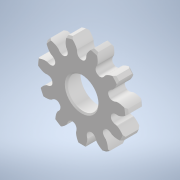
# Autodesk Inventor part: parasit_gear
Saved by Autodesk Inventor 2022 (Build 260153000, 153)
## iProperties
Created: 2024-09-10
Part Number: parasit_gear
Material: Типовые
Document SubType Name: Modeling
Designer: Andrey
Density: 1 g/cm^3
Appearance: По умолчанию
Author: Andrey
Autodesk Inventor part; units mm, degrees
ref_plane "YZ Plane" through (0, 0, 0) normal (1, 0, 0) x (0, 1, 0)
ref_plane "XZ Plane" through (0, 0, 0) normal (0, 1, 0) x (-1, 0, 0)
ref_plane "XY Plane" through (0, 0, 0) normal (0, 0, 1) x (1, 0, 0)
sketch "Эскиз1" plane through (0, 0, 0) normal (0, 0, 1) x (1, 0, 0)
  spline S0 degree 3 poles (-3.0473, 12.5821) (-3.001, 12.5436) (-2.9083, 12.4667) (-2.7729, 12.3469) (-2.6403, 12.2241) (-2.511, 12.0979) (-2.385, 11.9683) (-2.2627, 11.8352) (-2.1444, 11.6986) (-2.0303, 11.5585) (-1.9208, 11.4147) (-1.8163, 11.2672) (-1.7175, 11.1159) (-1.6248, 10.9607) (-1.5393, 10.8014) (-1.462, 10.638) (-1.4063, 10.498) (-1.368, 10.3837) (-1.3532, 10.3253) (-1.3457, 10.2961) knots 0 0 0 0 0.018071 0.036141 0.054212 0.072283 0.090353 0.108424 0.126494 0.144565 0.162635 0.180705 0.198775 0.216845 0.234914 0.252983 0.271051 0.280085 0.289119 0.289119 0.289119 0.289119
  spline S1 degree 3 poles (-1.3457, 10.2961) (-1.3472, 10.2417) (-1.3501, 10.1328) (-1.344, 9.9695) (-1.3289, 9.8068) (-1.3048, 9.6452) (-1.2696, 9.4855) (-1.2292, 9.3555) (-1.1924, 9.2529) (-1.1592, 9.1783) (-1.1249, 9.1042) (-1.0848, 9.033) (-1.042, 8.9634) (-0.9953, 8.8964) (-0.9441, 8.8326) (-0.8892, 8.7721) (-0.8304, 8.7153) (-0.7677, 8.663) (-0.7014, 8.6152) (-0.6317, 8.5725) (-0.559, 8.5352) (-0.4833, 8.5042) (-0.4054, 8.4796) (-0.3259, 8.4608) (-0.245, 8.4486) (-0.1361, 8.4437) (0, 8.4477) (0.1361, 8.4437) (0.245, 8.4486) (0.3259, 8.4608) (0.4054, 8.4796) (0.4833, 8.5042) (0.559, 8.5352) (0.6317, 8.5725) (0.7014, 8.6152) (0.7677, 8.663) (0.8304, 8.7153) (0.8892, 8.7721) (0.9441, 8.8326) (0.9953, 8.8964) (1.042, 8.9634) (1.0848, 9.033) (1.1249, 9.1042) (1.1592, 9.1783) (1.1924, 9.2529) (1.2292, 9.3555) (1.2696, 9.4855) (1.3048, 9.6452) (1.3289, 9.8068) (1.344, 9.9695) (1.3501, 10.1328) (1.3472, 10.2417) (1.3457, 10.2961) knots 0 0 0 0 0.016332 0.032664 0.048995 0.065326 0.081656 0.097985 0.106151 0.114317 0.122483 0.130649 0.138814 0.14698 0.155147 0.163312 0.171478 0.179642 0.187807 0.195971 0.204138 0.212304 0.220467 0.228631 0.236798 0.244962 0.261294 0.277626 0.28579 0.293957 0.302121 0.310284 0.31845 0.326617 0.334781 0.342945 0.35111 0.359276 0.367441 0.375607 0.383774 0.391939 0.400105 0.408271 0.416437 0.424603 0.440931 0.457262 0.473593 0.489924 0.506256 0.522588 0.522588 0.522588 0.522588
  spline S2 degree 3 poles (1.3457, 10.2961) (1.3532, 10.3253) (1.368, 10.3837) (1.4063, 10.498) (1.462, 10.638) (1.5393, 10.8014) (1.6248, 10.9607) (1.7175, 11.1159) (1.8163, 11.2672) (1.9208, 11.4147) (2.0303, 11.5585) (2.1444, 11.6986) (2.2627, 11.8352) (2.385, 11.9683) (2.511, 12.0979) (2.6403, 12.2241) (2.7729, 12.3469) (2.9083, 12.4667) (3.001, 12.5436) (3.0473, 12.5821) knots 0 0 0 0 0.009034 0.018069 0.036136 0.054205 0.072274 0.090344 0.108414 0.126484 0.144554 0.162625 0.180695 0.198766 0.216836 0.234907 0.252978 0.271048 0.289119 0.289119 0.289119 0.289119
  circle A0 centre (0, 0) radius 8.4461 construction
  circle A1 centre (0, 0) radius 10.3366 construction
  circle A2 centre (0, 0) radius 11 construction
  circle A3 centre (0, 0) radius 12.9458
  point P0 (-2.9089, 12.466)
  point P1 (-2.7734, 12.3464)
  point P2 (-2.6409, 12.2235)
  point P3 (-2.5115, 12.0973)
  point P4 (-2.3856, 11.9677)
  point P5 (-2.2634, 11.8346)
  point P6 (-2.1451, 11.698)
  point P7 (-2.0311, 11.5578)
  point P8 (-1.9216, 11.414)
  point P9 (-1.8173, 11.2665)
  point P10 (-1.7185, 11.1152)
  point P11 (-1.626, 10.96)
  point P12 (-1.5407, 10.8007)
  point P13 (-1.4637, 10.6372)
  point P14 (-1.3972, 10.4692)
  point P15 (-1.3691, 10.3834)
  point P16 (-1.3484, 10.1328)
  point P17 (-1.3425, 9.9696)
  point P18 (-1.3274, 9.807)
  point P19 (-1.303, 9.6455)
  point P20 (-1.2674, 9.4861)
  point P21 (-1.2196, 9.33)
  point P22 (-1.1915, 9.2533)
  point P23 (-1.159, 9.1784)
  point P24 (-1.1239, 9.1047)
  point P25 (-1.0843, 9.0332)
  point P26 (-1.0413, 8.9638)
  point P27 (-0.9945, 8.8969)
  point P28 (-0.9435, 8.8332)
  point P29 (-0.8886, 8.7727)
  point P30 (-0.8298, 8.7161)
  point P31 (-0.7671, 8.6637)
  point P32 (-0.7008, 8.6161)
  point P33 (-0.6312, 8.5734)
  point P34 (-0.5585, 8.5362)
  point P35 (-0.4829, 8.5053)
  point P36 (-0.4051, 8.4806)
  point P37 (-0.3256, 8.4619)
  point P38 (-0.2448, 8.4501)
  point P39 (-0.1633, 8.4456)
  point P40 (0, 8.4461)
  point P41 (0.1633, 8.4456)
  point P42 (0.2448, 8.4501)
  point P43 (0.3256, 8.4619)
  point P44 (0.4051, 8.4806)
  point P45 (0.4829, 8.5053)
  point P46 (0.5585, 8.5362)
  point P47 (0.6312, 8.5734)
  point P48 (0.7008, 8.6161)
  point P49 (0.7671, 8.6637)
  point P50 (0.8298, 8.7161)
  point P51 (0.8886, 8.7727)
  point P52 (0.9435, 8.8332)
  point P53 (0.9945, 8.8969)
  point P54 (1.0413, 8.9638)
  point P55 (1.0843, 9.0332)
  point P56 (1.1239, 9.1047)
  point P57 (1.159, 9.1784)
  point P58 (1.1915, 9.2533)
  point P59 (1.2196, 9.33)
  point P60 (1.2674, 9.4861)
  point P61 (1.303, 9.6455)
  point P62 (1.3274, 9.807)
  point P63 (1.3425, 9.9696)
  point P64 (1.3484, 10.1328)
  point P65 (1.3691, 10.3834)
  point P66 (1.3972, 10.4692)
  point P67 (1.4637, 10.6372)
  point P68 (1.5407, 10.8007)
  point P69 (1.626, 10.96)
  point P70 (1.7185, 11.1152)
  point P71 (1.8173, 11.2665)
  point P72 (1.9216, 11.414)
  point P73 (2.0311, 11.5578)
  point P74 (2.1451, 11.698)
  point P75 (2.2634, 11.8346)
  point P76 (2.3856, 11.9677)
  point P77 (2.5115, 12.0973)
  point P78 (2.6409, 12.2235)
  point P79 (2.7734, 12.3464)
  point P80 (2.9089, 12.466)
  constraints: 4 centre point, 2 point on circle, 177 other
extrude "Выдавливание1" add sketch "Эскиз1" along normal blind 4.75
chamfer "Фаска2" distance 0.5 angle 45 2 edges at (-12.9458, 0, 4.75) (-12.9458, 0, 0)
sketch "Эскиз4" plane through (0, 0, 4.75) normal (0, 0, 1) x (1, 0, 0)
  spline S0 degree 3 poles (-3.0473, 12.5821) (-3.001, 12.5436) (-2.9083, 12.4667) (-2.7729, 12.3469) (-2.6403, 12.2241) (-2.511, 12.0979) (-2.385, 11.9683) (-2.2627, 11.8352) (-2.1444, 11.6986) (-2.0303, 11.5585) (-1.9208, 11.4147) (-1.8163, 11.2672) (-1.7175, 11.1159) (-1.6248, 10.9607) (-1.5393, 10.8014) (-1.462, 10.638) (-1.4063, 10.498) (-1.368, 10.3837) (-1.3532, 10.3253) (-1.3457, 10.2961) knots 0 0 0 0 0.018071 0.036141 0.054212 0.072283 0.090353 0.108424 0.126494 0.144565 0.162635 0.180705 0.198775 0.216845 0.234914 0.252983 0.271051 0.280085 0.289119 0.289119 0.289119 0.289119
  spline S1 degree 3 poles (-1.3457, 10.2961) (-1.3472, 10.2417) (-1.3501, 10.1328) (-1.344, 9.9695) (-1.3289, 9.8068) (-1.3048, 9.6452) (-1.2696, 9.4855) (-1.2292, 9.3555) (-1.1924, 9.2529) (-1.1592, 9.1783) (-1.1249, 9.1042) (-1.0848, 9.033) (-1.042, 8.9634) (-0.9953, 8.8964) (-0.9441, 8.8326) (-0.8892, 8.7721) (-0.8304, 8.7153) (-0.7677, 8.663) (-0.7014, 8.6152) (-0.6317, 8.5725) (-0.559, 8.5352) (-0.4833, 8.5042) (-0.4054, 8.4796) (-0.3259, 8.4608) (-0.245, 8.4486) (-0.1361, 8.4437) (0, 8.4477) (0.1361, 8.4437) (0.245, 8.4486) (0.3259, 8.4608) (0.4054, 8.4796) (0.4833, 8.5042) (0.559, 8.5352) (0.6317, 8.5725) (0.7014, 8.6152) (0.7677, 8.663) (0.8304, 8.7153) (0.8892, 8.7721) (0.9441, 8.8326) (0.9953, 8.8964) (1.042, 8.9634) (1.0848, 9.033) (1.1249, 9.1042) (1.1592, 9.1783) (1.1924, 9.2529) (1.2292, 9.3555) (1.2696, 9.4855) (1.3048, 9.6452) (1.3289, 9.8068) (1.344, 9.9695) (1.3501, 10.1328) (1.3472, 10.2417) (1.3457, 10.2961) knots 0 0 0 0 0.016332 0.032664 0.048995 0.065326 0.081656 0.097985 0.106151 0.114317 0.122483 0.130649 0.138814 0.14698 0.155147 0.163312 0.171478 0.179642 0.187807 0.195971 0.204138 0.212304 0.220467 0.228631 0.236798 0.244962 0.261294 0.277626 0.28579 0.293957 0.302121 0.310284 0.31845 0.326617 0.334781 0.342945 0.35111 0.359276 0.367441 0.375607 0.383774 0.391939 0.400105 0.408271 0.416437 0.424603 0.440931 0.457262 0.473593 0.489924 0.506256 0.522588 0.522588 0.522588 0.522588
  spline S2 degree 3 poles (1.3457, 10.2961) (1.3532, 10.3253) (1.368, 10.3837) (1.4063, 10.498) (1.462, 10.638) (1.5393, 10.8014) (1.6248, 10.9607) (1.7175, 11.1159) (1.8163, 11.2672) (1.9208, 11.4147) (2.0303, 11.5585) (2.1444, 11.6986) (2.2627, 11.8352) (2.385, 11.9683) (2.511, 12.0979) (2.6403, 12.2241) (2.7729, 12.3469) (2.9083, 12.4667) (3.001, 12.5436) (3.0473, 12.5821) knots 0 0 0 0 0.009034 0.018069 0.036136 0.054205 0.072274 0.090344 0.108414 0.126484 0.144554 0.162625 0.180695 0.198766 0.216836 0.234907 0.252978 0.271048 0.289119 0.289119 0.289119 0.289119
  circle A0 centre (0, 0) radius 8.4461 construction
  circle A1 centre (0, 0) radius 10.3366 construction
  circle A2 centre (0, 0) radius 11 construction
  circle A3 centre (0, 0) radius 12.9458
  point P0 (-2.9089, 12.466)
  point P1 (-2.7734, 12.3464)
  point P2 (-2.6409, 12.2235)
  point P3 (-2.5115, 12.0973)
  point P4 (-2.3856, 11.9677)
  point P5 (-2.2634, 11.8346)
  point P6 (-2.1451, 11.698)
  point P7 (-2.0311, 11.5578)
  point P8 (-1.9216, 11.414)
  point P9 (-1.8173, 11.2665)
  point P10 (-1.7185, 11.1152)
  point P11 (-1.626, 10.96)
  point P12 (-1.5407, 10.8007)
  point P13 (-1.4637, 10.6372)
  point P14 (-1.3972, 10.4692)
  point P15 (-1.3691, 10.3834)
  point P16 (-1.3484, 10.1328)
  point P17 (-1.3425, 9.9696)
  point P18 (-1.3274, 9.807)
  point P19 (-1.303, 9.6455)
  point P20 (-1.2674, 9.4861)
  point P21 (-1.2196, 9.33)
  point P22 (-1.1915, 9.2533)
  point P23 (-1.159, 9.1784)
  point P24 (-1.1239, 9.1047)
  point P25 (-1.0843, 9.0332)
  point P26 (-1.0413, 8.9638)
  point P27 (-0.9945, 8.8969)
  point P28 (-0.9435, 8.8332)
  point P29 (-0.8886, 8.7727)
  point P30 (-0.8298, 8.7161)
  point P31 (-0.7671, 8.6637)
  point P32 (-0.7008, 8.6161)
  point P33 (-0.6312, 8.5734)
  point P34 (-0.5585, 8.5362)
  point P35 (-0.4829, 8.5053)
  point P36 (-0.4051, 8.4806)
  point P37 (-0.3256, 8.4619)
  point P38 (-0.2448, 8.4501)
  point P39 (-0.1633, 8.4456)
  point P40 (0, 8.4461)
  point P41 (0.1633, 8.4456)
  point P42 (0.2448, 8.4501)
  point P43 (0.3256, 8.4619)
  point P44 (0.4051, 8.4806)
  point P45 (0.4829, 8.5053)
  point P46 (0.5585, 8.5362)
  point P47 (0.6312, 8.5734)
  point P48 (0.7008, 8.6161)
  point P49 (0.7671, 8.6637)
  point P50 (0.8298, 8.7161)
  point P51 (0.8886, 8.7727)
  point P52 (0.9435, 8.8332)
  point P53 (0.9945, 8.8969)
  point P54 (1.0413, 8.9638)
  point P55 (1.0843, 9.0332)
  point P56 (1.1239, 9.1047)
  point P57 (1.159, 9.1784)
  point P58 (1.1915, 9.2533)
  point P59 (1.2196, 9.33)
  point P60 (1.2674, 9.4861)
  point P61 (1.303, 9.6455)
  point P62 (1.3274, 9.807)
  point P63 (1.3425, 9.9696)
  point P64 (1.3484, 10.1328)
  point P65 (1.3691, 10.3834)
  point P66 (1.3972, 10.4692)
  point P67 (1.4637, 10.6372)
  point P68 (1.5407, 10.8007)
  point P69 (1.626, 10.96)
  point P70 (1.7185, 11.1152)
  point P71 (1.8173, 11.2665)
  point P72 (1.9216, 11.414)
  point P73 (2.0311, 11.5578)
  point P74 (2.1451, 11.698)
  point P75 (2.2634, 11.8346)
  point P76 (2.3856, 11.9677)
  point P77 (2.5115, 12.0973)
  point P78 (2.6409, 12.2235)
  point P79 (2.7734, 12.3464)
  point P80 (2.9089, 12.466)
  constraints: 4 centre point, 2 point on circle, 177 other
extrude "Выдавливание4" cut sketch "Эскиз4" against normal blind 4.8 contours A3 S2 S1 S0 picked at (-0.3026, 11.4761)
pattern_circular "Круговой массив3" count 11 over 360 about axis through (0, 0, 0) along (0, 0, 1) of "Выдавливание4"
sketch "Эскиз5" plane through (0, 0, 0) normal (0, 0, -1) x (-1, 0, 0)
  circle A0 centre (0, 0) radius 5.1
  dimension "d23" = 10.2
  constraints: 1 centre point, 1 coincident
  measures "d23" diameter of A0
extrude "Выдавливание5" cut sketch "Эскиз5" against normal blind 4.05
sketch "Эскиз6" plane through (0, 0, 4.75) normal (0, 0, 1) x (1, 0, 0)
  circle A0 centre (0, 0) radius 2.1
  circle A1 centre (0, 0) radius 4.4
  dimension "d26" = 4.2
  dimension "d27" = 8.8
  constraints: 2 centre point, 2 coincident
  measures "d26" diameter of A0
  measures "d27" diameter of A1
extrude "Выдавливание6" cut sketch "Эскиз6" against normal blind 4.05 contours A0 | A1
chamfer "Фаска3" distance 0.4 angle 45 1 edges at (-4.4, 0, 4.75)
